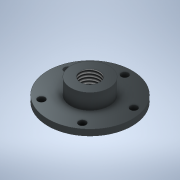
# Autodesk Inventor part: Part9
Saved by Autodesk Inventor 2020 (Build 240168000, 168)
## iProperties
Created: 2021-10-14
Part Number: Part9
Material: Iron, Cast
Document SubType Name: Modeling
Designer: simon.erikssonwestl
Density: 7.15 g/cm^3
Appearance: Iron Gray
Author: simon.erikssonwestl
Autodesk Inventor part; units mm, degrees
ref_plane "YZ Plane" through (0, 0, 0) normal (1, 0, 0) x (0, 1, 0)
ref_plane "XZ Plane" through (0, 0, 0) normal (0, 1, 0) x (-1, 0, 0)
ref_plane "XY Plane" through (0, 0, 0) normal (0, 0, 1) x (1, 0, 0)
sketch "Sketch1" plane through (0, 0, 0) normal (0, 1, 0) x (-1, 0, 0)
  circle A0 centre (0, 0) radius 17.5
  dimension "d0" = 35
  constraints: 1 centre point, 1 coincident
  measures "d0" diameter of A0
extrude "Extrusion1" add sketch "Sketch1" along normal mid plane 2.5
sketch "Sketch2" plane through (0, 1.25, 0) normal (0, 1, 0) x (1, 0, 0)
  circle A0 centre (0, 0) radius 8
  dimension "d3" = 16
  constraints: 1 centre point, 1 coincident
  measures "d3" diameter of A0
extrude "Extrusion2" add sketch "Sketch2" along normal blind 6.5
sketch "Sketch3" plane through (0, -1.25, 0) normal (0, -1, 0) x (1, 0, 0)
  circle A0 centre (0, 0) radius 9.5
  dimension "d6" = 19
  constraints: 1 centre point, 1 coincident
  measures "d6" diameter of A0
extrude "Extrusion3" add sketch "Sketch3" along normal blind 0.5
sketch "Sketch6" plane through (0, 1.25, 0) normal (0, 1, 0) x (1, 0, 0)
  circle A0 centre (0, 14.5) radius 1.5
  circle A1 centre (-13.7903, 4.4807) radius 1.5
  circle A2 centre (-8.5229, -11.7307) radius 1.5
  circle A3 centre (8.5229, -11.7307) radius 1.5
  circle A4 centre (13.7903, 4.4807) radius 1.5
  point P0 (0, 0)
  dimension "d17" = 3
  dimension "d18" = 14.5
  dimension "d21" = 360
  constraints: 5 centre point, 11 other
  measures "d17" diameter of A0
  measures "d18" distance of point (0, 0) A0.centre
extrude "Extrusion6" cut sketch "Sketch6" against normal through all
sketch "Sketch7" plane through (0, 7.75, 0) normal (0, 1, 0) x (1, 0, 0)
  point P0 (0, 0)
  point P1 (0, 0)
  constraints: 1 coincident
hole "Hole1" at (0, 7.75, 0) direction (0, -1, 0) diameter 8 depth 7 tip angle 118
sketch "Sketch8" plane through (0, -1.75, 0) normal (0, -1, 0) x (1, 0, 0)
  point P0 (0, 0)
hole "Hole2" at (0, -1.75, 0) direction (0, 1, 0) diameter 4 end through all
thread "Thread2" size "M8x1.25" class "6H" standard "ANSI Metric M Profile" full length
body "Solid1"
